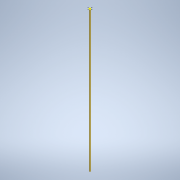
# Autodesk Inventor part: Tetrode
Saved by Autodesk Inventor 2020 (Build 240168000, 168)
## iProperties
Created: 2018-09-07
Part Number: Tetrode
Material: 일반
Document SubType Name: Modeling
Designer: Jeong Ji Hoon
Density: 1 g/cm^3
Appearance: 기본값
Author: Jeong Ji Hoon
Autodesk Inventor part; units mm, degrees
ref_plane "YZ Plane" through (0, 0, 0) normal (1, 0, 0) x (0, 1, 0)
ref_plane "XZ Plane" through (0, 0, 0) normal (0, 1, 0) x (-1, 0, 0)
ref_plane "XY Plane" through (0, 0, 0) normal (0, 0, 1) x (1, 0, 0)
sketch "Sketch2" plane through (0, 0, 0) normal (0, 0, 1) x (1, 0, 0)
  line L0 (0, 0) -> (0.1, 0) construction
  line L1 (0.1, 0) -> (0.1, 0.1)
  line L2 (0.1, 0.1) -> (0, 0.1) construction
  line L3 (0, 0.1) -> (0, 0) construction
  circle A0 centre (0.025, 0.075) radius 0.025
  circle A1 centre (0.075, 0.075) radius 0.025
  circle A2 centre (0.025, 0.025) radius 0.025
  circle A3 centre (0.075, 0.025) radius 0.025
  line L4 (0, 0.05) -> (0.1, 0.05)
  point P0 (0.05, 0.05)
  dimension "d11" = 0.1
  dimension "d12" = 0.1
  dimension "d13" = 0.05
  dimension "d14" = 0.05
  dimension "d16" = 0.05
  dimension "d18" = 0.05
  dimension "d22" = 0.05
  dimension "d23" = 0.05
  constraints: 10 end point, 8 tangent, 4 centre point, 2 midpoint, 2 parallel, 1 horizontal, 1 perpendicular
  measures "d11" distance of L2.end L1.end
  measures "d12" distance of L1.end L0.end
  measures "d13" diameter of A0
  measures "d14" diameter of A1
  measures "d16" diameter of A2
  measures "d18" diameter of A3
  measures "d22" distance from line of L3 point (0.05, 0.05)
  measures "d23" distance from line of L2 point (0.05, 0.05)
extrude "Extrusion1" add sketch "Sketch2" along normal blind 17 contours A3 | A2 | A1 | A0
sketch "스케치3" plane through (0, 0, 17) normal (0, 0, 1) x (1, 0, 0)
  arc A0 (0.05, 0.025) -> (0.025, 0.05) centre (0.025, 0.025) ccw construction
  arc A1 (0.025, 0.05) -> (0.05, 0.025) centre (0.025, 0.025) ccw construction
  arc A2 (0.05, 0.075) -> (0.025, 0.05) centre (0.025, 0.075) ccw construction
  arc A3 (0.025, 0.05) -> (0.05, 0.075) centre (0.025, 0.075) ccw construction
  arc A4 (0.075, 0.05) -> (0.05, 0.075) centre (0.075, 0.075) ccw construction
  arc A5 (0.05, 0.075) -> (0.075, 0.05) centre (0.075, 0.075) ccw construction
  arc A6 (0.05, 0.025) -> (0.075, 0.05) centre (0.075, 0.025) ccw construction
  arc A7 (0.075, 0.05) -> (0.05, 0.025) centre (0.075, 0.025) ccw construction
  arc A8 (0.025, 0.05) -> (0.05, 0.075) centre (0.025, 0.075) ccw construction
  arc A9 (0.05, 0.075) -> (0.075, 0.05) centre (0.075, 0.075) ccw construction
  line L0 (0.025, 0.05) -> (0.075, 0.05) construction
  point P0 (0, 0)
  point P1 (0.05, 0.05)
  constraints: 2 end point, 2 tangent, 1 horizontal, 1 midpoint
equation "\"d13\" = 0.5 * d12"
equation "\"d14\" = 0.5 * d15"
equation "\"d16\" = 0.5 * d17"
equation "\"d18\" = 0.5 * d19"
equation "\"d15\" = 0.1"
equation "\"d17\" = 0.1"
equation "\"d19\" = 0.1"
body "Solid1"
